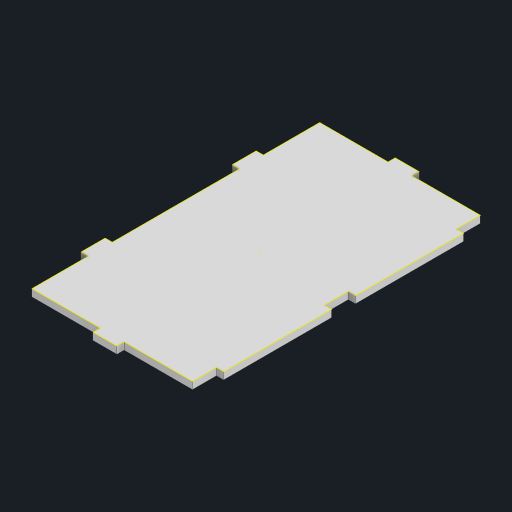
# Autodesk Inventor part: Bottom
Saved by Autodesk Inventor 2023 (Build 270158000, 158)
## iProperties
Created: 2024-07-21
Part Number: Bottom
Material: Generic
Document SubType Name: Modeling
Designer: Orsted
Density: 1 g/cm^3
Appearance: Default
Author: Orsted
Autodesk Inventor part; units mm, degrees
ref_plane "YZ Plane" through (0, 0, 0) normal (1, 0, 0) x (0, 1, 0)
ref_plane "XZ Plane" through (0, 0, 0) normal (0, 1, 0) x (-1, 0, 0)
ref_plane "XY Plane" through (0, 0, 0) normal (0, 0, 1) x (1, 0, 0)
sketch "Sketch1" plane through (0, 0, 0) normal (0, 1, 0) x (-1, 0, 0)
  line L0 (-35, -60) -> (35, -60)
  line L1 (35, -60) -> (35, 60)
  line L2 (35, 60) -> (-35, 60)
  line L3 (-35, 60) -> (-35, -60)
  line L4 (-35, -60) -> (35, 60) construction
  line L5 (35, -60) -> (-35, 60) construction
  point P0 (0, 0)
  dimension "d0" = 70
  dimension "d1" = 120
  constraints: 12 end point, 2 midpoint, 2 parallel, 1 horizontal, 1 perpendicular
  measures "d0" distance of L2.end L1.end
  measures "d1" distance of L0.end L1.end
extrude "Extrusion1" add sketch "Sketch1" along normal blind 3
sketch "Sketch2" plane through (0, 3, 0) normal (0, 1, 0) x (1, 0, 0)
  line L0 (35, -60) -> (32, -60)
  line L1 (32, -60) -> (32, -50)
  line L2 (32, -50) -> (35, -50)
  line L3 (35, -50) -> (35, -60)
  line L4 (35, -5) -> (32, -5)
  line L5 (32, -5) -> (32, 5)
  line L6 (32, 5) -> (35, 5)
  line L7 (35, 5) -> (35, -5)
  line L8 (35, 50) -> (32, 50)
  line L9 (32, 50) -> (32, 60)
  line L10 (32, 60) -> (35, 60)
  line L11 (35, 60) -> (35, 50)
  line L12 (35, -60) -> (35, 60) projected
  point P0 (0, 0)
  point P1 (35, 0)
  dimension "d4" = 3
  dimension "d5" = 10
  dimension "d6" = 3
  dimension "d7" = 10
  dimension "d8" = 10
  constraints: 24 end point, 6 parallel, 3 horizontal, 3 perpendicular, 2 midpoint, 2 point on line, 1 coincident
  measures "d4" distance of L1.end L2.end
  measures "d5" distance of L0.end L1.end
  measures "d6" distance of L5.end L6.end
  measures "d7" distance of L4.end L5.end
  measures "d8" distance of L8.end L9.end
extrude "Extrusion2" cut sketch "Sketch2" against normal through all
sketch "Sketch3" plane through (0, 0, 0) normal (0, -1, 0) x (1, 0, 0)
  line L0 (32, -60) -> (-35, -60) projected
  line L1 (3.5, 63) -> (-6.5, 63)
  line L2 (-6.5, 63) -> (-6.5, 60)
  line L3 (-6.5, 60) -> (3.5, 60)
  line L4 (3.5, 60) -> (3.5, 63)
  line L5 (3.5, -60) -> (-6.5, -60)
  line L6 (-6.5, -60) -> (-6.5, -63)
  line L7 (-6.5, -63) -> (3.5, -63)
  line L8 (3.5, -63) -> (3.5, -60)
  line L9 (-35, -60) -> (-35, 60) projected
  line L10 (-35, 60) -> (-25, 60)
  line L11 (-25, 60) -> (-25, 63)
  line L12 (-25, 63) -> (-35, 63)
  line L13 (-35, 63) -> (-35, 60)
  line L14 (-35, -60) -> (-25, -60)
  line L15 (-25, -60) -> (-25, -63)
  line L16 (-25, -63) -> (-35, -63)
  line L17 (-35, -63) -> (-35, -60)
  point P0 (0, 0)
  point P1 (32, 60)
  point P2 (-1.5, 60)
  point P3 (-1.5, -60)
  dimension "d15" = 10
  dimension "d16" = 3
  dimension "d17" = 10
  dimension "d18" = 3
  dimension "d21" = 10
  dimension "d22" = 10
  constraints: 32 end point, 8 parallel, 4 horizontal, 4 perpendicular, 3 midpoint
  measures "d15" distance of L3.end L2.end
  measures "d16" distance of L2.end L1.end
  measures "d17" distance of L7.end L6.end
  measures "d18" distance of L6.end L5.end
  measures "d21" distance of L12.end L11.end
  measures "d22" distance of L15.end L16.end
extrude "Extrusion3" add sketch "Sketch3" against normal blind 3 contours L8 L7 L6 L0 | L4 L3 L2 L1
sketch "Sketch4" plane through (0, 0, 0) normal (0, -1, 0) x (1, 0, 0)
  line L0 (-38, -36.5) -> (-35, -36.5)
  line L1 (-35, -36.5) -> (-35, -26.5)
  line L2 (-35, -26.5) -> (-38, -26.5)
  line L3 (-38, -26.5) -> (-38, -36.5)
  line L4 (-38, 26.5) -> (-35, 26.5)
  line L5 (-35, 26.5) -> (-35, 36.5)
  line L6 (-35, 36.5) -> (-38, 36.5)
  line L7 (-38, 36.5) -> (-38, 26.5)
  line L8 (-35, -60) -> (-35, 60) projected
  point P0 (0, 0)
  point P1 (-35, -31.5)
  point P2 (-35, -63)
  point P3 (-35, 63)
  point P4 (-35, 31.5)
  point P5 (-35, 0)
  point P6 (-35, 0)
  dimension "d23" = 3
  dimension "d24" = 10
  dimension "d25" = 3
  dimension "d26" = 10
  dimension "d27" = 126
  dimension "d28" = 31.5
  dimension "d29" = 31.5
  constraints: 16 end point, 4 midpoint, 4 parallel, 2 horizontal, 2 perpendicular, 2 point on line
  measures "d23" distance of L2.end L1.end
  measures "d24" distance of L1.end L0.end
  measures "d25" distance of L6.end L5.end
  measures "d26" distance of L5.end L4.end
  measures "d27" distance of point (-35, -63) point (-35, 63)
  measures "d28" distance of point (-35, 0) point (-35, -31.5)
  measures "d29" distance of point (-35, 0) point (-35, 31.5)
extrude "Extrusion4" add sketch "Sketch4" against normal blind 3
sketch "Sketch5" plane through (0, 3, 0) normal (0, 1, 0) x (1, 0, 0)
  line L0 (35, -50) -> (32, -50) projected
  line L1 (32, -50) -> (32, -60) projected
  line L2 (32, -60) -> (3.5, -60) projected
  line L3 (3.5, -60) -> (3.5, -63) projected
  line L4 (3.5, -63) -> (-6.5, -63) projected
  line L5 (-6.5, -63) -> (-6.5, -60) projected
  line L6 (-6.5, -60) -> (-35, -60) projected
  line L7 (-35, -60) -> (-35, -36.5) projected
  line L8 (-35, -36.5) -> (-38, -36.5) projected
  line L9 (-38, -36.5) -> (-38, -26.5) projected
  line L10 (-38, -26.5) -> (-35, -26.5) projected
  line L11 (-35, -26.5) -> (-35, 26.5) projected
  line L12 (-35, 26.5) -> (-38, 26.5) projected
  line L13 (-38, 26.5) -> (-38, 36.5) projected
  line L14 (-38, 36.5) -> (-35, 36.5) projected
  line L15 (-35, 36.5) -> (-35, 60) projected
  line L16 (-35, 60) -> (-6.5, 60) projected
  line L17 (-6.5, 60) -> (-6.5, 63) projected
  line L18 (-6.5, 63) -> (3.5, 63) projected
  line L19 (3.5, 63) -> (3.5, 60) projected
  line L20 (3.5, 60) -> (32, 60) projected
  line L21 (32, 60) -> (32, 50) projected
  line L22 (32, 50) -> (35, 50) projected
  line L23 (35, 50) -> (35, 5) projected
  line L24 (35, 5) -> (32, 5) projected
  line L25 (32, 5) -> (32, -5) projected
  line L26 (32, -5) -> (35, -5) projected
  line L27 (35, -5) -> (35, -50) projected
  point P0 (0, 0)
equation "\"d28\" = 0.25 * d27"
equation "\"d29\" = d28"
body "Solid1"
